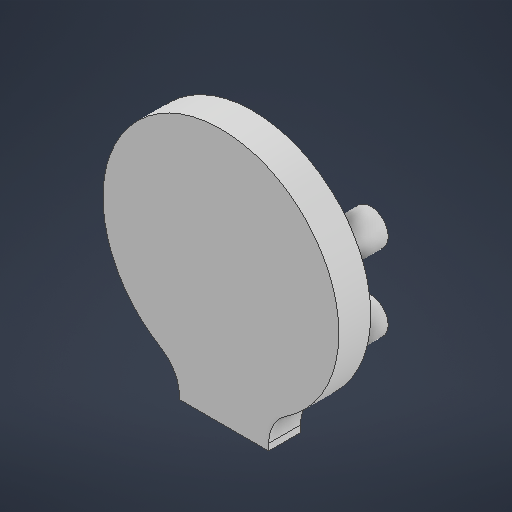
# Autodesk Inventor part: Disp
Saved by Autodesk Inventor 2026 (Build 300175000, 175)
## iProperties
Created: 2025-06-20
Part Number: Disp
Material: Všeobecné
Document SubType Name: Modeling
Designer: vadim
Density: 1 g/cm^3
Appearance: Výchozí
Author: vadim
Autodesk Inventor part; units mm, degrees
ref_plane "YZ Plane" through (0, 0, 0) normal (1, 0, 0) x (0, 1, 0)
ref_plane "XZ Plane" through (0, 0, 0) normal (0, 1, 0) x (-1, 0, 0)
ref_plane "XY Plane" through (0, 0, 0) normal (0, 0, 1) x (1, 0, 0)
sketch "Náčrt1" plane through (0, 0, 0) normal (0, 0, 1) x (1, 0, 0)
  arc A0 (10.1858, -15.4434) -> (-9.4468, -15.9062) centre (0, 0) ccw
  line L0 (7.4894, -20.4521) -> (7.4894, -21.5)
  line L1 (7.4894, -21.5) -> (-6.5106, -21.5)
  line L2 (-6.5106, -21.5) -> (-6.5106, -21.065)
  line L3 (0, -18.5) -> (7.4894, -21.5) construction
  line L4 (0, -18.5) -> (-6.5106, -21.5) construction
  line L5 (0, 18.5) -> (0, -37.4433)
  arc A1 (-6.5106, -21.065) -> (-9.4468, -15.9062) centre (-12.5106, -21.065) ccw
  arc A2 (10.1858, -15.4434) -> (7.4894, -20.4521) centre (13.4894, -20.4521) ccw
  line L6 (-12.5, 6) -> (12.5, 6)
  line L7 (12.5, 6) -> (12.5, -6)
  line L8 (12.5, -6) -> (-12.5, -6)
  line L9 (-12.5, -6) -> (-12.5, 6)
  line L10 (-12.5, 6) -> (12.5, -6) construction
  line L11 (12.5, 6) -> (-12.5, -6) construction
  circle A3 centre (-12.5, 6) radius 1.5
  circle A4 centre (12.5, 6) radius 1.5
  circle A5 centre (12.5, -6) radius 1.5
  circle A6 centre (-12.5, -6) radius 1.5
  circle A7 centre (-12.5, 6) radius 2.75
  circle A8 centre (12.5, 6) radius 2.75
  circle A9 centre (12.5, -6) radius 2.75
  circle A10 centre (-12.5, -6) radius 2.75
  point P0 (7.4894, -16.9162)
  point P1 (-6.5106, -17.3165)
  dimension "d0" = 37
  dimension "d1" = 14
  dimension "d2" = 21.5
  dimension "d3" = 6
  dimension "d4" = 25
  dimension "d5" = 12
  dimension "d6" = 3
  dimension "d7" = 3
  dimension "d8" = 3
  dimension "d9" = 3
  dimension "d10" = 5.5
  dimension "d11" = 5.5
  dimension "d12" = 5.5
  dimension "d13" = 5.5
  constraints: 24 end point, 11 centre point, 9 point on circle, 4 parallel, 4 point on line, 4 tangent, 3 coincident, 2 midpoint, 1 equal radius, 1 horizontal, 1 perpendicular
  measures "d0" diameter of A0
  measures "d1" distance of L0.end L1.end
  measures "d2" distance from line of A0.centre L1
  measures "d3" radius of A1
  measures "d4" distance of L7.end L8.end
  measures "d5" distance of L6.end L7.end
  measures "d6" diameter of A3
  measures "d7" diameter of A4
  measures "d8" diameter of A5
  measures "d9" diameter of A6
  measures "d10" diameter of A7
  measures "d11" diameter of A8
  measures "d12" diameter of A9
  measures "d13" diameter of A10
extrude "Vysunutí1" add sketch "Náčrt1" along normal blind 5
extrude "Vysunutí2" add sketch "Náčrt1" against normal blind 6 contours A7 L9 A3 L6 | L6 A3 L9 A7 | A8 L7 A4 L6 | L6 A4 L7 A8 | A9 L7 A5 L8 | L8 A5 L7 A9 | A10 L9 A6 L8 | L8 A6 L9 A10
thread "Závit1" size "M3x0.5" class "6H" standard "ISO Metric profile" full length
thread "Závit2" size "M3x0.5" class "6H" standard "ISO Metric profile" full length
thread "Závit3" size "M3x0.5" class "6H" standard "ISO Metric profile" full length
thread "Závit4" size "M3x0.5" class "6H" standard "ISO Metric profile" full length
